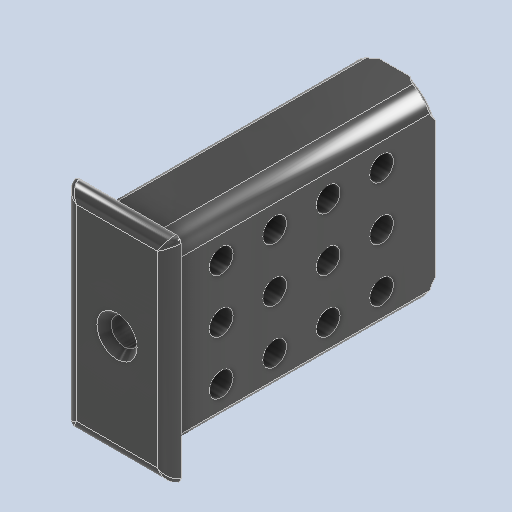
# Autodesk Inventor part: PLUG,MAXTUBE,2IN,3DP,TOP,ELEVATOR
Saved by Autodesk Inventor 2025.2 (Build 292293000, 293)
## iProperties
ILogicPurgeVersion: 0.0.0.0
OnSaveVersion: 3.4.3.0
OnSaveAssembly: COREAutomationManager
Created: 2025-02-06
Part Number: PLUG,MAXTUBE,2IN,3DP,TOP,ELEVATOR
Material: Nylon 6/6
Document SubType Name: Modeling
Designer: Jthib
Density: 1.13 g/cm^3
Appearance: Dark Gray
Mfg Approved By: John.Thibert
Mass: 54.0061 g
Surface Area: 143.213 cm^2
Volume: 47.793 cm^3
ModelCat: Uncategorized
MaterialName: Nylon 6/6
CN_MASS: 0.05
Author: Jthib
Autodesk Inventor part; units mm, degrees
ref_plane "YZ Plane" through (0, 0, 0) normal (1, 0, 0) x (0, 1, 0)
ref_plane "XZ Plane" through (0, 0, 0) normal (0, 1, 0) x (-1, 0, 0)
ref_plane "XY Plane" through (0, 0, 0) normal (0, 0, 1) x (1, 0, 0)
sketch "Sketch1" plane through (0, 0, 0) normal (0, 0, 1) x (1, 0, 0)
  arc A0 (-9.9442, -17.6598) -> (-4.9598, -22.6442) centre (0, -12.7) ccw construction
  line L0 (-4.8895, -24.257) -> (-4.8895, -22.7579) construction
  line L1 (-2.5, -24.384) -> (-0.127, -24.384) construction
  line L2 (-2.5, -24.384) -> (-4.7625, -24.384) construction
  arc A1 (-4.8895, -24.257) -> (-4.7625, -24.384) centre (-4.7625, -24.257) ccw construction
  arc A2 (-4.8895, -22.7579) -> (-4.9598, -22.6442) centre (-5.0165, -22.7579) ccw construction
  arc A3 (-9.9442, -17.6598) -> (-10.0579, -17.5895) centre (-10.0579, -17.7165) ccw construction
  line L3 (-10.0579, -17.5895) -> (-11.557, -17.5895) construction
  arc A4 (-11.684, -17.4625) -> (-11.557, -17.5895) centre (-11.557, -17.4625) ccw construction
  line L4 (-11.684, -17.4625) -> (-11.684, -15.2) construction
  line L5 (-11.684, -12.827) -> (-11.684, -15.2) construction
  line L6 (-11.684, -10.2) -> (-11.684, -12.573) construction
  line L7 (-11.684, -0.127) -> (-11.684, -2.5) construction
  line L8 (0, -24.257) -> (-4.7625, -24.257)
  line L9 (-4.7625, -24.257) -> (-4.7625, -22.7579)
  arc A5 (-4.7625, -22.7579) -> (-4.9031, -22.5306) centre (-5.0165, -22.7579) ccw
  arc A6 (-9.8306, -17.6031) -> (-4.9031, -22.5306) centre (0, -12.7) ccw
  arc A7 (-9.8306, -17.6031) -> (-10.0579, -17.4625) centre (-10.0579, -17.7165) ccw
  line L10 (-10.0579, -17.4625) -> (-11.557, -17.4625)
  line L11 (-11.557, -17.4625) -> (-11.557, -15.2)
  line L12 (-11.557, -15.2) -> (-11.557, 0)
  line L13 (0, 0) -> (-11.557, 0) construction
  line L14 (0, 24.257) -> (-4.7625, 24.257)
  line L15 (-4.7625, 24.257) -> (-4.7625, 22.7579)
  arc A8 (-4.9031, 22.5306) -> (-4.7625, 22.7579) centre (-5.0165, 22.7579) ccw
  arc A9 (-4.9031, 22.5306) -> (-9.8306, 17.6031) centre (0, 12.7) ccw
  arc A10 (-10.0579, 17.4625) -> (-9.8306, 17.6031) centre (-10.0579, 17.7165) ccw
  line L16 (-10.0579, 17.4625) -> (-11.557, 17.4625)
  line L17 (-11.557, 17.4625) -> (-11.557, 15.2)
  line L18 (-11.557, 15.2) -> (-11.557, 0)
  line L19 (0, 33.9905) -> (0, -34.1438) construction
  line L20 (0, -24.257) -> (4.7625, -24.257)
  line L21 (4.7625, -24.257) -> (4.7625, -22.7579)
  arc A11 (4.9031, -22.5306) -> (4.7625, -22.7579) centre (5.0165, -22.7579) ccw
  arc A12 (4.9031, -22.5306) -> (9.8306, -17.6031) centre (0, -12.7) ccw
  arc A13 (10.0579, -17.4625) -> (9.8306, -17.6031) centre (10.0579, -17.7165) ccw
  line L22 (10.0579, -17.4625) -> (11.557, -17.4625)
  line L23 (11.557, -17.4625) -> (11.557, -15.2)
  line L24 (11.557, -15.2) -> (11.557, 0)
  line L25 (0, 24.257) -> (4.7625, 24.257)
  line L26 (4.7625, 24.257) -> (4.7625, 22.7579)
  arc A14 (4.7625, 22.7579) -> (4.9031, 22.5306) centre (5.0165, 22.7579) ccw
  arc A15 (9.8306, 17.6031) -> (4.9031, 22.5306) centre (0, 12.7) ccw
  arc A16 (9.8306, 17.6031) -> (10.0579, 17.4625) centre (10.0579, 17.7165) ccw
  line L27 (10.0579, 17.4625) -> (11.557, 17.4625)
  line L28 (11.557, 17.4625) -> (11.557, 15.2)
  line L29 (11.557, 15.2) -> (11.557, 0)
  dimension "d0" = 0.127
  constraints: 58 end point, 36 symmetric about line, 34 point on circle, 17 centre point, 5 vertical, 4 horizontal, 1 vertical alignment, 52 other
  measures "d0" distance between parallel lines of L2 L8
extrude "Extrusion1" add sketch "Sketch1" against normal blind 63.5
sketch "Sketch2" plane through (0, 0, 0) normal (0, 0, 1) x (1, 0, 0)
  line L0 (12.7, 25.4) -> (-12.7, 25.4)
  line L1 (-12.7, 25.4) -> (-12.7, -25.4)
  line L2 (-12.7, -25.4) -> (12.7, -25.4)
  line L3 (12.7, -25.4) -> (12.7, 25.4)
  line L4 (12.7, 25.4) -> (-12.7, -25.4) construction
  line L5 (-12.7, 25.4) -> (12.7, -25.4) construction
  point P0 (0, 0)
  dimension "d3" = 25.4
  dimension "d4" = 50.8
  constraints: 12 end point, 2 midpoint, 2 parallel, 1 horizontal, 1 perpendicular
  measures "d3" distance of L2.end L1.end
  measures "d4" distance of L1.end L0.end
extrude "Extrusion2" add sketch "Sketch2" along normal blind 2.54
fillet "Fillet1" radius 3.175 4 edges at (-12.7, 0, 2.54) (0, -25.4, 2.54) (12.7, 0, 2.54) (0, 25.4, 2.54)
fillet "Fillet2" radius 1.27 4 edges at (-11.5972, 24.2972, 1.8243) (11.5972, 24.2972, 1.8243) (11.5972, -24.2972, 1.8243) (-11.5972, -24.2972, 1.8243)
sketch "Sketch3" plane through (0, 0, 2.54) normal (0, 0, 1) x (1, 0, 0)
  point P0 (0, 0)
  point P1 (0, 0)
  constraints: 1 coincident
hole "Hole1" at (0, 0, 2.54) direction (0, 0, -1) diameter 6.35 end through all countersink diameter 9.525 countersink angle 82
sketch "Sketch4" plane through (-11.557, -17.4625, -63.5) normal (-1, 0, 0) x (0, 0, 1)
  line L0 (50.8, 4.7625) -> (50.8, 30.1625) construction
  line L1 (63.5, 51.4223) -> (63.5, -16.4973) construction
  line L2 (63.5, 34.925) -> (63.5, 0) construction
  point P0 (63.5, 17.4625)
  point P1 (50.8, 17.4625)
  point P2 (63.5, 17.4625)
  dimension "d26" = 12.7
  dimension "d27" = 25.4
  constraints: 2 coincident, 2 end point, 2 midpoint, 1 horizontal alignment, 1 parallel
  measures "d26" distance between parallel lines of L1 L0
  measures "d27" distance of L0.start L0.end
hole "Hole2" at (-11.557, -12.7, -12.7) at (-11.557, 0, -12.7) at (-11.557, 12.7, -12.7) direction (1, 0, 0) diameter 5.6134 end through all clearance for "Flat Head Machine Screw (82)" size "#10" standard "Ansi Unified Screw Threads"
chamfer "Chamfer1" distance 1.27 angle 45 24 edges at (-11.557, 0, -63.5) (-7.7679, -20.4679, -63.5) (-9.9242, -17.5005, -63.5) (-10.8074, -17.4625, -63.5) (-4.8005, -22.6242, -63.5) (-4.7625, -23.5074, -63.5) (7.7679, -20.4679, -63.5) (4.8005, -22.6242, -63.5) (4.7625, -23.5074, -63.5) (9.9242, -17.5005, -63.5) (10.8074, -17.4625, -63.5) (0, -24.257, -63.5) (11.557, 0, -63.5) (7.7679, 20.4679, -63.5) (9.9242, 17.5005, -63.5) (10.8074, 17.4625, -63.5) (4.8005, 22.6242, -63.5) (4.7625, 23.5074, -63.5) (0, 24.257, -63.5) (-7.7679, 20.4679, -63.5) (-4.8005, 22.6242, -63.5) (-4.7625, 23.5074, -63.5) (-9.9242, 17.5005, -63.5) (-10.8074, 17.4625, -63.5)
pattern_linear "Rectangular Pattern1" count 4 spacing 12.7 along (0, 0, -1) of "Hole2"
sketch "Sketch5" plane through (0, 0, -63.5) normal (0, 0, -1) x (-1, 0, 0)
  line L0 (12.7, -25.4) -> (-12.7, -25.4)
  line L1 (-12.7, -25.4) -> (-12.7, 25.4)
  line L2 (-12.7, 25.4) -> (12.7, 25.4)
  line L3 (12.7, 25.4) -> (12.7, -25.4)
  line L4 (12.7, -25.4) -> (-12.7, 25.4) construction
  line L5 (-12.7, -25.4) -> (12.7, 25.4) construction
  line L6 (-9.525, 22.225) -> (-9.525, -22.225)
  line L7 (-9.525, -22.225) -> (9.525, -22.225)
  line L8 (9.525, -22.225) -> (9.525, 22.225)
  line L9 (9.525, 22.225) -> (-9.525, 22.225)
  point P0 (0, 0)
  dimension "d31" = 25.4
  dimension "d32" = 50.8
  dimension "d33" = 3.175
  constraints: 20 end point, 4 parallel, 2 midpoint, 2 perpendicular, 1 horizontal, 3 other
  measures "d31" distance of L1.end L2.end
  measures "d32" distance of L0.end L1.end
  measures "d33" distance between parallel lines of L1 L6
extrude "Extrusion3" cut sketch "Sketch5" against normal up to surface (63.5 mm away)
body "Solid1"
